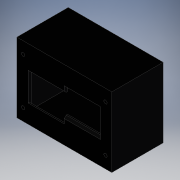
# Autodesk Inventor part: GA06
Saved by Autodesk Inventor 2017 (Build 210142000, 142)
## iProperties
Created: 2018-11-17
Part Number: GA06
Material: ABS Plastic
Document SubType Name: Modeling
Designer: Dell
Density: 1.06 g/cm^3
Appearance: Smooth - Black
Author: Dell
Autodesk Inventor part; units mm, degrees
ref_plane "YZ Plane" through (0, 0, 0) normal (1, 0, 0) x (0, 1, 0)
ref_plane "XZ Plane" through (0, 0, 0) normal (0, 1, 0) x (-1, 0, 0)
ref_plane "XY Plane" through (0, 0, 0) normal (0, 0, 1) x (1, 0, 0)
sketch "Sketch1" plane through (0, 0, 0) normal (0, 0, 1) x (1, 0, 0)
  line L0 (0, 0) -> (0, 70) construction
  circle A0 centre (0, 0) radius 2.5
  circle A1 centre (0, 70) radius 2.5
  line L1 (0, 0) -> (125, 0) construction
  circle A2 centre (125, 0) radius 2.5
  circle A3 centre (125, 70) radius 2.5
  line L2 (-7.5, -16) -> (132.5, -16)
  line L3 (132.5, -16) -> (132.5, 86)
  line L4 (132.5, 86) -> (-7.5, 86)
  line L5 (-7.5, 86) -> (-7.5, -16)
  point P0 (62.5, 0)
  point P1 (62.5, -16)
  point P2 (0, 35)
  point P3 (-7.5, 35)
  dimension "d0" = 70
  dimension "d1" = 5
  dimension "d2" = 5
  dimension "d3" = 5
  dimension "d4" = 5
  dimension "d5" = 125
  dimension "d6" = 140
  dimension "d7" = 102
  constraints: 12 end point, 4 centre point, 4 midpoint, 3 coincident, 2 horizontal, 2 horizontal alignment, 2 parallel, 2 vertical alignment, 1 perpendicular, 1 vertical
  measures "d0" distance of L0.start L0.end
  measures "d1" diameter of A0
  measures "d2" diameter of A1
  measures "d3" diameter of A2
  measures "d4" diameter of A3
  measures "d5" distance of L1.start L1.end
  measures "d6" distance of L4.end L3.end
  measures "d7" distance of L3.end L2.end
extrude "Extrusion1" add sketch "Sketch1" along normal blind 5
sketch "Sketch2" plane through (0, 0, 5) normal (0, 0, 1) x (1, 0, 0)
  line L0 (7.5, 60) -> (117.5, 60)
  line L1 (117.5, 60) -> (117.5, 10)
  line L2 (117.5, 10) -> (7.5, 10)
  line L3 (7.5, 10) -> (7.5, 60)
  line L4 (-7.5, 86) -> (-7.5, -16) projected
  line L5 (132.5, 86) -> (-7.5, 86) projected
  point P0 (0, 0)
  point P1 (62.5, 60)
  point P2 (62.5, 86)
  point P3 (7.5, 35)
  point P4 (-7.5, 35)
  dimension "d10" = 15
  dimension "d11" = 50
  constraints: 8 end point, 4 midpoint, 2 parallel, 1 horizontal, 1 horizontal alignment, 1 perpendicular, 1 vertical alignment
  measures "d10" distance between parallel lines of L4 L3
  measures "d11" distance of L0.end L1.end
extrude "Extrusion2" cut sketch "Sketch2" against normal through all
sketch "Sketch3" plane through (-7.5, 86, 0) normal (0, 1, 0) x (1, 0, 0)
  line L0 (140, 0) -> (140, -5) projected
  line L1 (140, -5) -> (0, -5)
  line L2 (0, -5) -> (0, 73)
  line L3 (0, 73) -> (140, 73)
  line L4 (140, 73) -> (140, -5)
  point P0 (7.5, 0)
  dimension "d17" = 78
  constraints: 8 end point, 2 parallel, 1 coincident, 1 horizontal, 1 perpendicular
  measures "d17" distance of L1.end L2.end
extrude "Extrusion3" add sketch "Sketch3" along normal blind 2
sketch "Sketch4" plane through (-7.5, -16, 0) normal (0, -1, 0) x (1, 0, 0)
  line L0 (140, 0) -> (0, 0) projected
  line L1 (0, 0) -> (0, -73) projected
  line L2 (0, -73) -> (140, -73) projected
  line L3 (140, -73) -> (140, 0) projected
  line L4 (0, 0) -> (140, 0) projected
  line L5 (140, 0) -> (140, 5) projected
  line L6 (0, 5) -> (140, 5) projected
  line L7 (0, 0) -> (0, 5) projected
  point P0 (7.5, 0)
extrude "Extrusion4" add sketch "Sketch4" along normal blind 2
sketch "Sketch5" plane through (-7.5, 86, -73) normal (-1, 0, 0) x (0, 0, 1)
  line L0 (78, -104) -> (78, 2) projected
  line L1 (0, -102) -> (0, -104) projected
  line L2 (78, 2) -> (0, 2)
  line L3 (0, 2) -> (0, -104)
  line L4 (0, -104) -> (78, -104)
  line L5 (78, -104) -> (78, 2)
  point P0 (73, -86)
  constraints: 8 end point, 2 parallel, 1 horizontal, 1 perpendicular
extrude "Extrusion5" add sketch "Sketch5" along normal blind 2
sketch "Sketch6" plane through (132.5, 86, 0) normal (1, 0, 0) x (0, 0, -1)
  line L0 (-5, -104) -> (-5, 2) projected
  line L1 (-5, -104) -> (73, -104)
  line L2 (73, -104) -> (73, 2)
  line L3 (73, 2) -> (-5, 2)
  line L4 (-5, 2) -> (-5, -104)
  point P0 (0, -86)
  constraints: 8 end point, 2 parallel, 1 horizontal, 1 perpendicular
extrude "Extrusion6" add sketch "Sketch6" along normal blind 2
sketch "Sketch7" plane through (0, 0, 5) normal (0, 0, 1) x (1, 0, 0)
  line L0 (117.5, 10) -> (7.5, 10) construction
  line L1 (7.5, 60) -> (117.5, 60) construction
  line L2 (7.5, 10) -> (7.5, 60) construction
  line L3 (117.5, 60) -> (117.5, 10) construction
  line L4 (7.5, 60) -> (62.5, 60)
  line L5 (62.5, 60) -> (62.5, 50)
  line L6 (62.5, 50) -> (7.5, 50)
  line L7 (7.5, 50) -> (7.5, 60)
  line L8 (117.5, 10) -> (62.5, 10)
  line L9 (62.5, 10) -> (62.5, 20)
  line L10 (62.5, 20) -> (117.5, 20)
  line L11 (117.5, 20) -> (117.5, 10)
  line L12 (117.5, 10) -> (7.5, 10) projected
  line L13 (7.5, 60) -> (117.5, 60) projected
  line L14 (7.5, 10) -> (7.5, 60) projected
  point P0 (0, 0)
  point P1 (62.5, 10)
  point P2 (7.5, 35)
  dimension "d26" = 55
  dimension "d27" = 10
  dimension "d28" = 55
  dimension "d29" = 10
  constraints: 24 end point, 6 midpoint, 4 parallel, 2 horizontal, 2 perpendicular
  measures "d26" distance of L5.end L6.end
  measures "d27" distance of L4.end L5.end
  measures "d28" distance of L9.end L10.end
  measures "d29" distance of L8.end L9.end
extrude "Extrusion7" add sketch "Sketch7" against normal blind 5
chamfer "Chamfer2" distance 3 angle 45 4 edges at (35, 10, 0) (90, 60, 0) (90, 20, 5) (35, 50, 5)
body "Solid1"
